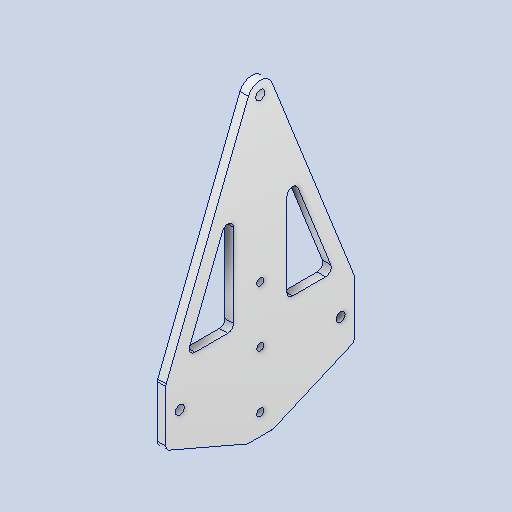
# Autodesk Inventor part: odom_v1_Plate_6
Saved by Autodesk Inventor 2025.2 (Build 292293000, 293)
## iProperties
Created: 2025-04-02
Part Number: odom_v1_Plate_6
Material: アルミニウム 6061
Document SubType Name: Modeling
Designer: haruy
Density: 2.7 g/cm^3
Appearance: アルミニウム - フラット
Author: haruy
Autodesk Inventor part; units mm, degrees
ref_plane "YZ Plane" through (0, 0, 0) normal (1, 0, 0) x (0, 1, 0)
ref_plane "XZ Plane" through (0, 0, 0) normal (0, 1, 0) x (-1, 0, 0)
ref_plane "XY Plane" through (0, 0, 0) normal (0, 0, 1) x (1, 0, 0)
derived "odom_v1_Sketch_Base.ipt"
sketch "スケッチ1" plane through (300, 0, 0) normal (1, 0, 0) x (0, 1, 0)
  line L0 (0, 0) -> (20, 0)
  line L1 (20, 0) -> (20, -192.6893)
  line L2 (20, -192.6893) -> (0, -192.6893)
  line L3 (0, -192.6893) -> (0, 0)
  line L4 (-77, 0) -> (-77, -265.1297)
  circle A0 centre (7.5, -57.9764) radius 1.6
  circle A1 centre (7.5, -93.4764) radius 1.6
  line L5 (-20, -52.2264) -> (-66, -52.2264)
  line L6 (-66, -52.2264) -> (-66, -57.2264)
  line L7 (-66, -57.2264) -> (-20, -57.2264)
  line L8 (-20, -57.2264) -> (-20, -52.2264)
  line L9 (-20, -94.2264) -> (-66, -94.2264)
  line L10 (-66, -94.2264) -> (-66, -99.2264)
  line L11 (-66, -99.2264) -> (-20, -99.2264)
  line L12 (-20, -99.2264) -> (-20, -94.2264)
  line L13 (-19.371, -66.7264) -> (-77, -66.7264)
  line L14 (-77, -66.7264) -> (-77, -84.7264)
  line L15 (-77, -84.7264) -> (-19.371, -84.7264)
  line L16 (-19.371, -84.7264) -> (-19.371, -66.7264)
  line L17 (-41.1855, -57.2264) -> (-55.1855, -57.2264)
  line L18 (-55.1855, -57.2264) -> (-55.1855, -58.0264)
  line L19 (-55.1855, -58.0264) -> (-41.1855, -58.0264)
  line L20 (-41.1855, -58.0264) -> (-41.1855, -57.2264)
  line L21 (-48.1855, -66.7264) -> (-48.1855, -84.7264)
  line L22 (-55.1855, -94.2264) -> (-41.1855, -94.2264)
  line L23 (-41.1855, -94.2264) -> (-41.1855, -93.4264)
  line L24 (-41.1855, -93.4264) -> (-55.1855, -93.4264)
  line L25 (-55.1855, -93.4264) -> (-55.1855, -94.2264)
  circle A2 centre (48, -75.7264) radius 1.65
  circle A3 centre (-17, -75.7264) radius 2
  line L26 (48, -75.7264) -> (-17, -75.7264)
  line L27 (33.5, -67.2264) -> (-12, -67.2264)
  line L28 (-12, -67.2264) -> (-12, -84.2264)
  line L29 (-12, -84.2264) -> (33.5, -84.2264)
  line L30 (33.5, -84.2264) -> (33.5, -67.2264)
  line L31 (-12, -73.7264) -> (-20, -73.7264)
  line L32 (-20, -73.7264) -> (-20, -77.7264)
  line L33 (-20, -77.7264) -> (-12, -77.7264)
  line L34 (-12, -77.7264) -> (-12, -73.7264)
  line L35 (-2, -71.2264) -> (-57, -71.2264)
  line L36 (-57, -71.2264) -> (-57, -80.2264)
  line L37 (-57, -80.2264) -> (-2, -80.2264)
  line L38 (-2, -80.2264) -> (-2, -71.2264)
  circle A4 centre (-9.5, -75.7264) radius 1.25
  circle A5 centre (-29.5, -75.7264) radius 1.25
  circle A6 centre (-49.5, -75.7264) radius 1.25
  line L39 (-52, -65.7264) -> (-22, -65.7264)
  line L40 (-22, -65.7264) -> (-22, -85.7264)
  line L41 (-22, -85.7264) -> (-52, -85.7264)
  line L42 (-52, -85.7264) -> (-52, -65.7264)
  line L43 (-43, -52.2264) -> (-43, -57.2264)
  circle A7 centre (-33, -54.7264) radius 1.5
  line L44 (-29.5, -75.7264) -> (-49.5, -75.7264)
  circle A8 centre (-53, -54.7264) radius 1.5
  circle A9 centre (-53, -96.7264) radius 1.5
  circle A10 centre (-33, -96.7264) radius 1.5
  line L45 (-44.5, -42.2264) -> (-24.5, -42.2264)
  line L46 (-24.5, -42.2264) -> (-24.5, -168.1987)
  line L47 (-24.5, -168.1987) -> (-44.5, -168.1987)
  line L48 (-44.5, -168.1987) -> (-44.5, -42.2264)
  circle A11 centre (-34.5, -47.2264) radius 1.6
  circle A12 centre (48, -75.7264) radius 4.5
  line L49 (-2, -71.2264) -> (48, -71.2264)
  line L50 (-2, -80.2264) -> (1.4883, -80.2264)
  line L51 (1.4883, -80.2264) -> (48, -80.2264)
  circle A13 centre (-34.5, -104.2264) radius 1.6
  line L52 (-44.5, -109.2264) -> (-24.5, -109.2264)
  line L53 (-24.5, -42.2264) -> (49.6544, -71.5416)
  line L54 (-44.5, -42.2264) -> (-57, -71.2264)
  line L55 (-26.3382, -46.8763) -> (47.8162, -76.1914)
  line L56 (-19.5, -42.2264) -> (-19.5, -173.1987)
  line L57 (-19.5, -173.1987) -> (-49.5, -173.1987)
  line L58 (-49.5, -173.1987) -> (-49.5, -42.2264)
  line L59 (-1.9528, -66.2264) -> (48, -66.2264)
  line L60 (-1.9528, -66.2264) -> (-19.5, -66.2264)
  line L61 (-24.5, -109.2264) -> (49.6544, -79.9113)
  line L62 (-44.5, -109.2264) -> (-57, -80.2264)
  line L63 (-26.3382, -104.5766) -> (47.8162, -75.2614)
  line L64 (-1.9528, -85.2264) -> (48, -85.2264)
  line L65 (-1.9528, -85.2264) -> (-19.5, -85.2264)
  point P0 (-24.5, -71.2264)
  point P1 (-44.5, -71.2264)
  point P2 (-44.5, -80.2264)
  point P3 (-24.5, -80.2264)
  point P4 (-19.5, -101.8733)
  point P5 (22.6092, -85.2264)
  point P6 (-19.371, -80.2264)
  point P7 (-19.5, -84.7264)
  point P8 (-19.5, -80.2264)
  point P9 (-19.5, -71.2264)
  point P10 (-19.5, -66.7264)
  point P11 (-19.371, -71.2264)
  point P12 (22.6092, -66.2264)
  point P13 (-19.5, -49.5796)
  dimension "d1" = 20
  dimension "d3" = 32.5
  dimension "d4" = 3.2
  dimension "d5" = 5
  dimension "d6" = 10
  dimension "d7" = 5
  dimension "d8" = 9
  dimension "d11" = 5
  dimension "d12" = 5
  dimension "d13" = 5
  measures "d1" distance of L46.end L47.end
  measures "d3" distance between parallel lines of L4 L48
  measures "d4" diameter of A11
  measures "d5" distance from line of L45 A11.centre
  measures "d6" distance from line of A11.centre L48
  measures "d7" distance from line of L5 A11.centre
  measures "d8" diameter of A12
  measures "d11" distance between parallel lines of L53 L55
  measures "d12" distance between parallel lines of L46 L56
  measures "d13" distance between parallel lines of L49 L59
extrude "押し出し1" add sketch "スケッチ1" against normal blind 3 contours L53 L1 L55 L3 | L3 L55 L56 L53 | L53 L59 L55 L1 | L56 L55 L46 L53 | L53 A12 L49 L55 L30 L27 L59 | L59 L1 L27 L3 | L3 L27 L28 L35 L16 L13 L56 L60 L59 | L56 L13 L40 L39 L46 L7 L8 L5 L55 | L46 L5 L48 L45 | L59 L55 L27 L1 | A12 L63 A2 L55 | L27 L1 L49 L3 | L3 L49 L35 L28 L27 | L48 L5 L54 | L27 L55 L30 L49 L1 | L27 L30 L55 | A12 L55 L49 | L49 L1 L26 L3 | L3 L26 L38 L49 | L46 L7 L43 L5 | L5 L8 L7 L46 | L56 L35 L40 L13 | L13 L16 L35 L56 | L48 L7 L58 L54 L5 | L5 L43 L7 L48 | L49 L30 L26 L1 | L55 L49 L30 | L61 L64 L63 L29 L30 L51 A12 | L55 A2 L26 A12 | A12 L26 L30 L49 L55 | L26 L1 L51 L50 L3 | L3 L50 L38 L26 | L38 L26 A4 L28 L35 | L28 L31 L16 L35 | L46 L39 L48 L19 L20 L7 | L40 L35 L46 L13 | L13 L46 L39 L40 | L56 L31 L32 L33 L37 L40 L35 | L35 L16 L31 L56 | L48 L19 L58 L7 | L7 L20 L19 L48 | L58 L7 L54 | L26 L30 L51 L1 | L51 L63 A12 | L61 L1 L63 L64 | A12 L63 L51 L30 L26 | L26 A2 L63 A12 | L50 L51 L1 L29 L3 | L3 L29 L28 L37 L50 | L38 L37 L28 L26 A4 | L28 L26 A3 L31 | L46 L13 L48 L39 | L46 L35 L48 L13 | L40 L37 L46 L35 | L56 L33 L32 L31 | L31 L16 L33 L56 | L58 L19 L54 L7 | L48 L39 L58 L19 | L51 L30 L63 L29 L1 | L63 L30 L51 | L61 L3 L63 L1 | L64 L1 L29 L63 | L29 L1 L64 L3 | L3 L64 L65 L56 L15 L16 L37 L28 L29 | L28 L33 A3 L26 | A3 | A3 L33 L16 L31 | L48 L13 L58 L39 | L48 L35 L21 L13 | L46 L37 L48 L35 | L40 L15 L46 L37 | L37 L56 L15 L40 | L33 L16 L37 L56 | L58 L39 L42 L13 L54 L19 | L30 L29 L63 | L61 L56 L63 L3 | L37 L16 L33 L28 | L58 L13 L42 L39 | L21 L35 L58 L13 | L48 L44 L21 L35 | L46 L15 L48 L37 | L37 L16 L15 L56 | L40 L41 L46 L15 | L15 L56 L63 L46 L11 L12 L9 L41 L40 | L13 L42 L35 L54 | L61 L46 L63 L56 | L58 L35 L42 L13 | L21 L44 A6 L58 L35 | L48 L37 L21 L44 | L48 L15 L21 L37 | L46 L41 L48 L15 | L35 L42 L37 L36 | L52 L48 L11 L46 | L58 A6 L37 L42 L35 | L21 L37 L58 A6 L44 | L21 L15 L58 L37 | L48 L41 L58 L15 | L46 L9 L23 L24 L48 L41 | L37 L42 L15 L62 | L62 L11 L48 | L58 L15 L42 L37 | L48 L24 L58 L41 | L46 L11 L48 L9 | L9 L12 L11 L46 | L15 L42 L41 L58 L24 L62 | L11 L62 L58 L9 L48 | L58 L41 L42 L15 | L48 L9 L58 L24 | L24 L23 L9 L48 | L24 L58 L9 L62 | L62 L9 L58 | A0 | A1 | A7 | A10
fillet "フィレット1" radius 2 12 edges at (298.5, -19.5, -49.5796) (298.5, -19.5, -66.2264) (298.5, 22.6092, -66.2264) (298.5, 22.6092, -85.2264) (298.5, -19.5, -85.2264) (298.5, -19.5, -101.8733) (298.5, -24.5, -109.2264) (298.5, -44.5, -109.2264) (298.5, -57, -80.2264) (298.5, -57, -71.2264) (298.5, -44.5, -42.2264) (298.5, -24.5, -42.2264)
